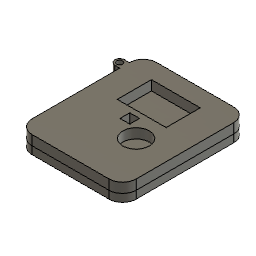
TiltCase (Autodesk Fusion 360 design; units mm, degrees)
Autodesk Fusion 360 part; units mm, degrees
sketch "Sketch1" plane through (0, 0, 0) normal (0, 1, 0) x (1, 0, 0)
  line L0 (-28, 40) -> (7.4, 40)
  line L1 (14.4, 33) -> (14.4, -12.9)
  line L2 (7.4, -19.9) -> (-28, -19.9)
  line L3 (-35, -12.9) -> (-35, 33)
  arc A0 (14.4, 33) -> (7.4, 40) centre (7.4, 33) ccw
  arc A1 (7.4, -19.9) -> (14.4, -12.9) centre (7.4, -12.9) ccw
  arc A2 (-28, 40) -> (-35, 33) centre (-28, 33) ccw
  arc A3 (-35, -12.9) -> (-28, -19.9) centre (-28, -12.9) ccw
  line L4 (-30, 42) -> (9.4, 42)
  line L5 (16.4, 35) -> (16.4, -14.9)
  line L6 (9.4, -21.9) -> (-30, -21.9)
  line L7 (-37, -14.9) -> (-37, 35)
  arc A4 (-30, 42) -> (-37, 35) centre (-30, 35) ccw
  arc A5 (16.4, 35) -> (9.4, 42) centre (9.4, 35) ccw
  arc A6 (9.4, -21.9) -> (16.4, -14.9) centre (9.4, -14.9) ccw
  arc A7 (-37, -14.9) -> (-30, -21.9) centre (-30, -14.9) ccw
  point P0 (-35, 40)
  point P1 (14.4, 40)
  point P2 (-35, -19.9)
  dimension "d1" = 59.9
  dimension "d2" = 49.4
  dimension "d3" = 7
  dimension "d4" = 7
  dimension "d5" = 7
  dimension "d6" = 7
  dimension "d7" = 2
  dimension "d8" = 2
  dimension "d9" = 2
  dimension "d10" = 2
  dimension "d11" = 7
  dimension "d12" = 7
  dimension "d13" = 7
  dimension "d14" = 7
  constraint horizontal L0
  constraint vertical L1
  constraint horizontal L2
  constraint vertical L3
  constraint coincident P1 L0
  constraint coincident P1 L1
  constraint tangent L0 A0
  constraint tangent L1 A0
  constraint tangent L2 A1
  constraint tangent L1 A1
  constraint coincident P0 L0
  constraint coincident P0 L3
  constraint tangent L0 A2
  constraint tangent L3 A2
  constraint coincident P2 L3
  constraint coincident P2 L2
  constraint tangent L3 A3
  constraint tangent L2 A3
  constraint horizontal L4
  constraint vertical L5
  constraint horizontal L6
  constraint vertical L7
  constraint tangent L4 A4
  constraint tangent L7 A4
  constraint tangent L4 A5
  constraint tangent L5 A5
  constraint tangent L6 A6
  constraint tangent L5 A6
  constraint tangent L7 A7
  constraint tangent L6 A7
  measures "d1" distance of P0 P2
  measures "d2" distance of P0 P1
  measures "d3" radius of A0
  measures "d4" radius of A1
  measures "d5" radius of A2
  measures "d6" radius of A3
  measures "d7" distance of L0 L4
  measures "d8" distance of L1 L5
  measures "d9" distance of L3 L7
  measures "d10" distance of L2 L6
  measures "d11" radius of A4
  measures "d12" radius of A5
  measures "d13" radius of A6
  measures "d14" radius of A7
extrude "Extrude1" add sketch "Sketch1" along normal blind 2 contours L0 L1 L2 L3 A0 A1 A2 A3 makes body 1
extrude "Extrude2" add sketch "Sketch1" along normal blind 4 bodies 1
sketch "Sketch2" plane through (0, 0, 21.9) normal (0, 0, 1) x (1, 0, 0)
  line L0 (-30, 0) -> (9.4, 0)
  line L1 (9.4, 0) -> (9.4, 4)
  line L2 (9.4, 4) -> (-30, 4)
  line L3 (-30, 4) -> (-30, 0)
  line L4 (-27, 8) -> (-18, 8)
  line L5 (-18, 8) -> (-18, 4.5)
  line L6 (-18, 4.5) -> (-27, 4.5)
  line L7 (-27, 4.5) -> (-27, 8)
  line L8 (9.4, 0) -> (-30, 0)
  dimension "d19" = 9
  dimension "d20" = 3.5
  dimension "d21" = 4.5
  dimension "d22" = 3
  constraint horizontal L4
  constraint vertical L5
  constraint horizontal L6
  constraint vertical L7
  measures "d19" distance of L4.start L4.end
  measures "d20" distance of L4.start L6.end
  measures "d21" distance of L6 L8
  measures "d22" distance of L3 L7
sketch "Sketch5" plane through (0, 2, 0) normal (0, 1, 0) x (-1, 0, 0)
  arc A0 (28, -40) -> (35, -33) centre (28, -33) ccw
  line L0 (35, -33) -> (35, 12.9)
  arc A1 (35, 12.9) -> (28, 19.9) centre (28, 12.9) ccw
  line L1 (28, 19.9) -> (-7.4, 19.9)
  arc A2 (-7.4, 19.9) -> (-14.4, 12.9) centre (-7.4, 12.9) ccw
  line L2 (-14.4, 12.9) -> (-14.4, -33)
  arc A3 (-14.4, -33) -> (-7.4, -40) centre (-7.4, -33) ccw
  line L3 (-7.4, -40) -> (28, -40)
  line L4 (23.75, -33) -> (-1.25, -33)
  line L5 (-1.25, -33) -> (-1.25, -15.5)
  line L6 (-1.25, -15.5) -> (23.75, -15.5)
  line L7 (23.75, -15.5) -> (23.75, -33)
  line L8 (14.6, -12.75) -> (9.6, -12.75)
  line L9 (9.6, -12.75) -> (9.6, -7.75)
  line L10 (9.6, -7.75) -> (14.6, -7.75)
  line L11 (14.6, -7.75) -> (14.6, -12.75)
  line L12 (-14.4, -33) -> (-14.4, 12.9)
  line L13 (28, -40) -> (-7.4, -40)
  line L14 (35, 12.9) -> (35, -33)
  circle A4 centre (1.6, -3) radius 6.75
  line L15 (30, -42) -> (-9.4, -42)
  line L16 (-16.4, -35) -> (-16.4, 14.9)
  line L17 (-9.4, 21.9) -> (30, 21.9)
  line L18 (37, 14.9) -> (37, -35)
  line L19 (-7.4, 19.9) -> (28, 19.9)
  arc A5 (30, -42) -> (37, -35) centre (30, -35) ccw
  arc A6 (-16.4, -35) -> (-9.4, -42) centre (-9.4, -35) ccw
  arc A7 (-9.4, 21.9) -> (-16.4, 14.9) centre (-9.4, 14.9) ccw
  arc A8 (37, 14.9) -> (30, 21.9) centre (30, 14.9) ccw
  dimension "d34" = 25
  dimension "d35" = 5
  dimension "d36" = 5
  dimension "d37" = 24
  dimension "d39" = 17.5
  dimension "d41" = 7
  dimension "d42" = 27.25
  dimension "d43" = 11.25
  dimension "d47" = 13.5
  dimension "d48" = 37
  dimension "d49" = 16
  dimension "d53" = 2
  dimension "d54" = 2
  dimension "d55" = 2
  dimension "d56" = 2
  dimension "d57" = 7
  dimension "d58" = 7
  dimension "d59" = 7
  dimension "d60" = 7
  constraint horizontal L4
  constraint vertical L5
  constraint horizontal L6
  constraint vertical L7
  constraint horizontal L8
  constraint vertical L9
  constraint horizontal L10
  constraint vertical L11
  constraint horizontal L15
  constraint vertical L16
  constraint horizontal L17
  constraint vertical L18
  constraint tangent L15 A5
  constraint tangent L18 A5
  constraint tangent L15 A6
  constraint tangent L16 A6
  constraint tangent L17 A7
  constraint tangent L16 A7
  constraint tangent L17 A8
  constraint tangent L18 A8
  measures "d34" distance of L4.start L4.end
  measures "d35" distance of L8.end L9.end
  measures "d36" distance of L9.end L10.end
  measures "d37" distance of L9 L12
  measures "d39" distance of L4.start L6.end
  measures "d41" distance of L4 L13
  measures "d42" distance of L8 L13
  measures "d43" distance of L7 L14
  measures "d47" diameter of A4
  measures "d48" distance of L13 A4.centre
  measures "d49" distance of L12 A4.centre
  measures "d53" distance of L12 L16
  measures "d54" distance of L17 L19
  measures "d55" distance of L14 L18
  measures "d56" distance of L13 L15
  measures "d57" radius of A5
  measures "d58" radius of A6
  measures "d59" radius of A7
  measures "d60" radius of A8
extrude "Extrude8" add sketch "Sketch5" along normal blind 5 from surface at 2 separate body contours A0 L0 A1 L1 A2 L2 A3 L3 L12 L13 L14 L19 | L15 L16 L17 L18 A5 A6 A7 A8 makes body 2
sketch "Sketch10" plane through (-37, 0, 0) normal (-1, 0, 0) x (0, 0, 1)
  line L0 (-35, 4) -> (14.9, 4)
  line L1 (14.9, 4) -> (14.9, 9)
  line L2 (14.9, 9) -> (-35, 9)
  line L3 (-35, 9) -> (-35, 4)
  line L4 (-35, 9) -> (-30, 9)
  line L5 (-30, 9) -> (-30, 4)
  line L6 (-30, 4) -> (-35, 4)
  line L7 (-35, 4) -> (-35, 9)
  dimension "d80" = 5
  dimension "d81" = 5
  constraint horizontal L4
  constraint vertical L5
  constraint horizontal L6
  constraint vertical L7
  constraint coincident L2.end L3.start
  measures "d80" distance of L2.end L0.start
  measures "d81" distance of L2.end L4.end
extrude "Extrude13" add sketch "Sketch10" along normal blind 5 contours L0 L2 L3 L4 L5 L6 L7 bodies 2
sketch "Sketch11" plane through (0, 9, 0) normal (0, 1, 0) x (-1, 0, 0)
  line L0 (37, -35) -> (42, -35)
  line L1 (42, -35) -> (42, -30)
  line L2 (42, -30) -> (37, -30)
  line L3 (39.5, -35) -> (37, -35)
  line L4 (37, -35) -> (37, -30)
  line L5 (37, -30) -> (39.5, -30)
  circle A0 centre (39.5, -32.5) radius 1.5
  arc A1 (39.5, -35) -> (42, -32.5) centre (39.5, -32.5) ccw
  arc A2 (42, -32.5) -> (39.5, -30) centre (39.5, -32.5) ccw
  line L6 (-1.25, -15.5) -> (23.75, -15.5)
  line L7 (23.75, -15.5) -> (23.75, -33)
  line L8 (23.75, -33) -> (-1.25, -33)
  line L9 (-1.25, -33) -> (-1.25, -15.5)
  line L10 (9.6, -7.75) -> (14.6, -7.75)
  line L11 (14.6, -7.75) -> (14.6, -12.75)
  line L12 (14.6, -12.75) -> (9.6, -12.75)
  line L13 (9.6, -12.75) -> (9.6, -7.75)
  circle A3 centre (1.6, -3) radius 6.75
  arc A4 (30, -42) -> (37, -35) centre (30, -35) ccw
  line L14 (37, -30) -> (37, 14.9)
  arc A5 (37, 14.9) -> (30, 21.9) centre (30, 14.9) ccw
  line L15 (30, 21.9) -> (-9.4, 21.9)
  arc A6 (-9.4, 21.9) -> (-16.4, 14.9) centre (-9.4, 14.9) ccw
  line L16 (-16.4, 14.9) -> (-16.4, -35)
  arc A7 (-16.4, -35) -> (-9.4, -42) centre (-9.4, -35) ccw
  line L17 (-9.4, -42) -> (30, -42)
  dimension "d84" = 3
  dimension "d85" = 2.5
  dimension "d86" = 2.5
  constraint horizontal L3
  constraint vertical L4
  constraint horizontal L5
  constraint coincident L2.end L4.end
  constraint tangent L3 A1
  constraint tangent L5 A2
  constraint coincident A1.end A2.start
  measures "d84" diameter of A0
  measures "d85" radius of A1
  measures "d86" radius of A2
extrude "Extrude14" cut sketch "Sketch11" against normal blind 5 contours L0 L1 A1 | L1 L2 A2 | A0 bodies 1 2
equation "d1 = 59.5 mm + 0.4 mm"
equation "d2 = 49 mm + 0.4 mm"
equation "d41 = 2.2 mm + 4.8 mm"
equation "d43 = 8.75 mm + 2.5 mm"
named bodies: "Bottom", "Top"
